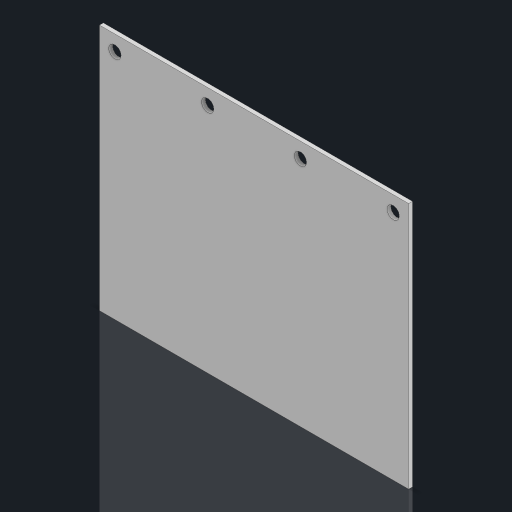
# Autodesk Inventor part: Polycarbonate Kicker plate
Saved by Autodesk Inventor 2023.2 (Build 272271030, 271C)
## iProperties
Created: 2023-12-10
Part Number: Polycarbonate Kicker plate
Material: Generic
Document SubType Name: Modeling
Designer: Michael
Density: 1 g/cm^3
Appearance: Default
Author: Michael
Autodesk Inventor part; units mm, degrees
ref_plane "YZ Plane" through (0, 0, 0) normal (1, 0, 0) x (0, 1, 0)
ref_plane "XZ Plane" through (0, 0, 0) normal (0, 1, 0) x (-1, 0, 0)
ref_plane "XY Plane" through (0, 0, 0) normal (0, 0, 1) x (1, 0, 0)
sketch "Sketch1" plane through (0, 0, 0) normal (0, 0, 1) x (1, 0, 0)
  line L0 (0, 0) -> (-127, 0)
  line L1 (-127, 0) -> (-127, 101.6)
  line L2 (-127, 101.6) -> (0, 101.6)
  line L3 (0, 101.6) -> (0, 0)
  dimension "d0" = 127
  dimension "d1" = 101.6
  constraints: 8 end point, 2 parallel, 1 horizontal, 1 perpendicular
  measures "d0" distance of L1.end L2.end
  measures "d1" distance of L0.end L1.end
extrude "Extrusion1" add sketch "Sketch1" along normal blind 1.5875
sketch "Sketch3" plane through (0, 0, 1.5875) normal (0, 0, 1) x (1, 0, 0)
  line L0 (0, 101.6) -> (-127, 101.6) projected
  line L1 (-6.35, 101.6) -> (-6.35, 95.25)
  line L2 (-6.35, 95.25) -> (0, 95.25)
  line L3 (0, 0) -> (0, 101.6) projected
  circle A0 centre (-6.35, 95.25) radius 2.54
  line L4 (-6.35, 95.25) -> (-44.45, 95.25)
  line L5 (-44.45, 95.25) -> (-82.55, 95.25)
  line L6 (-82.55, 95.25) -> (-120.65, 95.25)
  line L7 (-120.65, 95.25) -> (-127, 95.25)
  circle A1 centre (-44.45, 95.25) radius 2.54
  circle A2 centre (-82.55, 95.25) radius 2.54
  circle A3 centre (-120.65, 95.25) radius 2.54
  dimension "d4" = 6.35
  dimension "d5" = 6.35
  dimension "d6" = 5.08
  dimension "d7" = 38.1
  dimension "d8" = 38.1
  dimension "d9" = 38.1
  dimension "d10" = 6.35
  dimension "d11" = 5.08
  dimension "d12" = 5.08
  dimension "d13" = 5.08
  constraints: 12 end point, 5 point on line, 4 centre point, 4 coincident, 2 horizontal, 1 perpendicular
  measures "d4" distance of L1.start L1.end
  measures "d5" distance of L1.end L2.end
  measures "d6" diameter of A0
  measures "d7" distance of L4.start L4.end
  measures "d8" distance of L4.end L5.end
  measures "d9" distance of L5.end L6.end
  measures "d10" distance of L6.end L7.end
  measures "d11" diameter of A1
  measures "d12" diameter of A2
  measures "d13" diameter of A3
extrude "Extrusion2" cut sketch "Sketch3" against normal blind 25.4 contours A0 L2 L1 | L1 L4 A0 | A0 L4 L2 | A1 L5 L4 | L4 L5 A1 | A2 L6 L5 | L5 L6 A2 | A3 L7 L6 | L6 L7 A3
body "Solid1"
